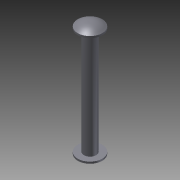
# Autodesk Inventor part: 02
Saved by Autodesk Inventor 2016 (Build 200138000, 138)
## iProperties
Created: 2014-01-27
Part Number: 02
Material: Generic
Document SubType Name: Modeling
Designer: Michał
Density: 1 g/cm^3
Appearance: Default
Author: Michał
Autodesk Inventor part; units mm, degrees
ref_plane "YZ Plane" through (0, 0, 0) normal (1, 0, 0) x (0, 1, 0)
ref_plane "XZ Plane" through (0, 0, 0) normal (0, 1, 0) x (-1, 0, 0)
sketch "Sketch1" plane through (0, 0, 0) normal (0, 0, 1) x (1, 0, 0)
  circle A0 centre (0, 0) radius 1
  dimension "d0" = 2
  constraints: 1 centre point, 1 coincident
  measures "d0" diameter of A0
extrude "Extrusion1" add sketch "Sketch1" along normal blind 17.5
sketch "Sketch2" plane through (0, 0, 17.5) normal (0, 0, 1) x (1, 0, 0)
  circle A0 centre (0, 0) radius 1 projected
  circle A1 centre (0, 0) radius 2
  dimension "d3" = 4
  constraints: 1 centre point, 1 coincident
  measures "d3" diameter of A1
extrude "Extrusion2" add sketch "Sketch2" along normal blind 1 contours A0 | A1
chamfer "Chamfer1" distance 0.7 distance2 1 1 edges at (-2, 0, 18.5) measured on face at (1.9935, -0.1609, 18.1667)
fillet "Fillet1" radius 2.75 1 edges at (-1, 0, 18.5)
ref_plane "Work Plane1" through (0, 0, 8.75) normal (0, 0, -1) x (-1, 0, 0)
mirror "Mirror1" about plane through (0, 0, 8.75) normal (0, 0, -1) of "Extrusion2", "Chamfer1", "Fillet1"
body "Solid1"
